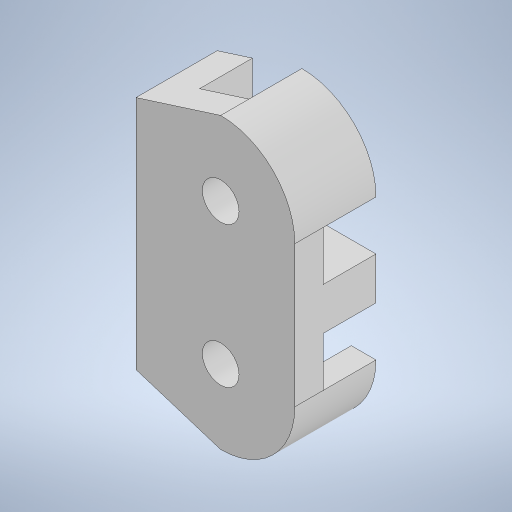
# Autodesk Inventor part: XZ Bearing Cage
Saved by Autodesk Inventor 2023.1 (Build 271208000, 208)
## iProperties
Created: 2022-12-02
Part Number: XZ Bearing Cage
Material: Generic
Document SubType Name: Modeling
Designer: nicol
Density: 1 g/cm^3
Appearance: Default
Author: nicol
Autodesk Inventor part; units mm, degrees
ref_plane "YZ Plane" through (0, 0, 0) normal (1, 0, 0) x (0, 1, 0)
ref_plane "XZ Plane" through (0, 0, 0) normal (0, 1, 0) x (-1, 0, 0)
ref_plane "XY Plane" through (0, 0, 0) normal (0, 0, 1) x (1, 0, 0)
sketch "Sketch1" plane through (0, 0, 0) normal (0, 0, 1) x (1, 0, 0)
  circle A0 centre (12, 30.5) radius 7
  circle A1 centre (12, 10.5) radius 7
  line L0 (5, 23.5) -> (22.5, 23.5)
  line L1 (22.5, 23.5) -> (22.5, 17.5)
  line L2 (22.5, 17.5) -> (5, 17.5)
  line L3 (5, 17.5) -> (5, 23.5)
  line L4 (0, 41) -> (5, 41)
  line L5 (5, 41) -> (5, 0)
  line L6 (5, 0) -> (0, 0)
  line L7 (0, 0) -> (0, 41)
  circle A2 centre (12, 10.5) radius 2.6
  circle A3 centre (12, 30.5) radius 2.6
  circle A4 centre (12, 30.5) radius 10.5
  circle A5 centre (12, 10.5) radius 10.5
  line L8 (5, 41) -> (12, 41)
  line L9 (22.5, 23.5) -> (22.5, 30.5)
  line L10 (22.5, 17.5) -> (22.5, 10.5)
  line L11 (5, 0) -> (12, 0)
  line L12 (12, 10.5) -> (12, 0)
  line L13 (12, 10.5) -> (22.5, 10.5)
  line L14 (12, 30.5) -> (12, 41)
  line L15 (12, 30.5) -> (22.5, 30.5)
  point P0 (5, 17.5)
  point P1 (5, 23.5)
  point P2 (5, 10.5)
  point P3 (12, 17.5)
  point P4 (5, 30.5)
  point P5 (12, 23.5)
  point P6 (19, 10.5)
  point P7 (12, 3.5)
  point P8 (19, 30.5)
  point P9 (12, 37.5)
  dimension "d0" = 20
  dimension "d1" = 14
  dimension "d2" = 5.2
  dimension "d3" = 5.2
  dimension "d6" = 3.5
  dimension "d13" = 5
  constraints: 32 end point, 7 perpendicular, 7 tangent, 6 centre point, 5 coincident, 4 parallel, 4 point on circle, 2 equal radius, 2 horizontal, 1 collinear, 1 point on line, 1 vertical, 1 vertical alignment
  measures "d0" distance of A1.centre A0.centre
  measures "d1" diameter of A0
  measures "d2" diameter of A2
  measures "d3" diameter of A3
  measures "d6" radial gap between concentric circles of A1 A5
  measures "d13" distance of L4.start L4.end
extrude "Extrusion1" add sketch "Sketch1" against normal blind 7.5 contours A0 L14 A4 L15 | L0 L5 A0 | L0 A4 A5 L3 | L5 L3 A4 | L0 L1 L2 A5 A4 | A4 L3 A5 L5 L6 L7 L4 | A4 A5 L3 | A5 L2 L3 A4 | A4 A5 | L3 L5 A5 | A5 L12 A1 L13 | L2 A1 L5
extrude "Extrusion2" add sketch "Sketch1" along normal blind 4 contours L15 A3 L14 A0 | L15 A4 L0 A0 | A0 L14 A3 L15 | A0 L14 A4 L15 | A0 L5 A4 L14 | L0 L5 A0 | L0 A4 A5 L3 | L9 L0 A4 | L5 L3 A4 | A4 L5 L8 | L0 L1 L2 A5 A4 | A4 L3 A5 L5 L6 L7 L4 | A4 A5 L3 | A5 L2 L3 A4 | A4 A5 | L10 A5 L2 | L3 L5 A5 | A5 L13 A1 L2 | A5 L12 A1 L13 | L2 A1 L5 | A5 L11 L5 | L5 A1 L12 A5 | A1 L13 A2 L12 | A1 L12 A2 L13
sketch "Sketch2" plane through (0, 0, 4) normal (0, 0, 1) x (1, 0, 0)
  line L0 (12, 41) -> (0, 41) projected
  line L1 (0, 41) -> (0, 0) projected
  line L2 (0, 0) -> (12, 0) projected
  arc A0 (12, 0) -> (22.5, 10.5) centre (12, 10.5) ccw projected
  line L3 (22.5, 10.5) -> (22.5, 30.5) projected
  arc A1 (22.5, 30.5) -> (12, 41) centre (12, 30.5) ccw projected
  circle A2 centre (12, 10.5) radius 2.6 projected
  circle A3 centre (12, 30.5) radius 2.6 projected
  arc A4 (22.5, 30.5) -> (12, 41) centre (12, 30.5) ccw projected
  line L4 (12, 41) -> (0, 37.1888)
  line L5 (5, 0) -> (12, 0) projected
  line L6 (12, 0) -> (0, 3.8112)
  dimension "d14" = 17.62
  constraints: 4 end point, 2 point on line, 1 equal length
  measures "d14" angle of L0 L4
extrude "Extrusion3" cut sketch "Sketch2" against normal through all contours L4 L1 L0 | L6 L2 L1
body "Solid1"
